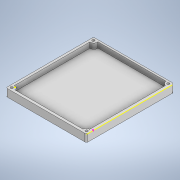
# Autodesk Inventor part: Case rev.1
Saved by Autodesk Inventor 2020.2 (Build 242310000, 310)
## iProperties
Created: 2019-11-25
Part Number: Case rev.1
Material: Generic
Document SubType Name: Modeling
Designer: athiy
Density: 1 g/cm^3
Appearance: Default
Author: athiy
Autodesk Inventor part; units mm, degrees
ref_plane "YZ Plane" through (0, 0, 0) normal (1, 0, 0) x (0, 1, 0)
ref_plane "XZ Plane" through (0, 0, 0) normal (0, 1, 0) x (-1, 0, 0)
ref_plane "XY Plane" through (0, 0, 0) normal (0, 0, 1) x (1, 0, 0)
sketch "Sketch1" plane through (0, 0, 0) normal (0, 1, 0) x (-1, 0, 0)
  line L0 (-81.2549, 4.894) -> (-81.2549, -88.547)
  line L1 (4.6415, -88.547) -> (4.6415, 4.894)
  line L2 (4.6415, -88.547) -> (-81.2549, -88.547)
  line L3 (4.6415, 4.894) -> (-81.2549, 4.894)
  point P0 (0, 0)
  dimension "d103" = 93.4411
  dimension "d104" = 85.8964
  constraints: 8 end point, 1 horizontal, 1 perpendicular, 1 vertical
  measures "d103" distance between parallel lines of L2 L3
  measures "d104" distance between parallel lines of L0 L1
extrude "Extrusion1" add sketch "Sketch1" along normal blind 8
fillet "Fillet1" radius 2 1 edges at (81.2549, 4, -88.547)
sketch "Sketch2" plane through (0, 8, 0) normal (0, 1, 0) x (1, 0, 0)
  point P0 (0, 0)
sketch "Sketch9" plane through (0, 8, 0) normal (0, 1, 0) x (1, 0, 0)
  line L0 (81.2549, -4.894) -> (81.2549, 86.547) projected
  point P0 (0, 0)
  point P1 (81.2549, 2)
sketch "Sketch15" plane through (0, 8, 0) normal (0, 1, 0) x (1, 0, 0)
  point P0 (0, 0)
sketch "Sketch16" plane through (0, 8, 0) normal (0, 1, 0) x (1, 0, 0)
  circle A0 centre (-0.8495, 85.0914) radius 1.27
  line L0 (-4.6415, 88.547) -> (-4.6415, -4.894) projected
  line L1 (81.2549, -4.894) -> (81.2549, 86.547) projected
  circle A1 centre (-0.8495, -1.4384) radius 1.27
  line L2 (-2.1195, 82.1131) -> (-2.1195, 1.3369)
  line L3 (2.1021, 86.547) -> (74.7894, 86.547)
  arc A2 (-2.1195, 82.1131) -> (2.1021, 86.547) centre (-1.6738, 85.9154) ccw
  line L4 (2.1021, -2.1183) -> (74.7894, -2.1183)
  line L5 (78.4154, 82.1131) -> (78.4154, 1.3369)
  arc A3 (74.7894, 86.547) -> (78.4154, 82.1131) centre (80.0457, 87.1459) ccw
  arc A4 (78.4154, 1.3369) -> (74.7894, -2.1183) centre (78.0984, -1.9607) ccw
  arc A5 (2.1021, -2.1183) -> (-2.1195, 1.3369) centre (-1.3126, -1.9838) ccw
  circle A6 centre (78.0984, -1.9607) radius 1.27
  circle A7 centre (78.0984, 85.6137) radius 1.27
  point P0 (0, 0)
  point P1 (79.2549, 88.547)
  constraints: 8 centre point, 8 end point, 8 point on circle, 2 horizontal, 1 coincident, 1 parallel, 1 vertical
extrude "Extrusion14" cut sketch "Sketch16" against normal blind 5.75 contours A2 L3 A3 L5 A4 L4 A5 L2
sketch "Sketch17" plane through (0, 8, 0) normal (0, 1, 0) x (1, 0, 0)
  circle A0 centre (-1.6277, -1.7597) radius 1.27
  line L0 (-4.6415, 88.547) -> (-4.6415, -4.894) projected
  line L1 (-4.6415, 41.8265) -> (80.9593, 41.8265)
  circle A1 centre (-1.6277, 85.4127) radius 1.27
  circle A2 centre (78.2293, -1.7597) radius 1.27
  circle A3 centre (78.2293, 85.4127) radius 1.27
  point P0 (0, 0)
  constraints: 4 centre point, 2 end point, 2 symmetric about line, 1 horizontal, 1 midpoint, 2 other
extrude "Extrusion15" cut sketch "Sketch17" against normal blind 2
fillet "Fillet4" radius 1.6 3 edges at (81.2549, 4, 4.894) (-4.6415, 4, -88.547) (-4.6415, 4, 4.894)
sketch "Sketch20" plane through (0, 2.25, 0) normal (0, 1, 0) x (1, 0, 0)
  point P0 (0, 0)
body "Solid1"
